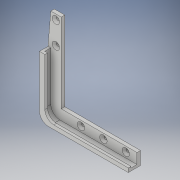
# Autodesk Inventor part: iPadGolf6HolderMount
Saved by Autodesk Inventor 2017 (Build 210142000, 142)
## iProperties
Created: 2022-11-14
Part Number: iPadGolf6HolderMount
Material: Generic
Document SubType Name: Modeling
Designer: khonsu
Density: 1 g/cm^3
Appearance: Default
Author: khonsu
Autodesk Inventor part; units mm, degrees
ref_plane "YZ Plane" through (0, 0, 0) normal (1, 0, 0) x (0, 1, 0)
ref_plane "XZ Plane" through (0, 0, 0) normal (0, 1, 0) x (-1, 0, 0)
ref_plane "XY Plane" through (0, 0, 0) normal (0, 0, 1) x (1, 0, 0)
sketch "Sketch1" plane through (0, 0, 0) normal (0, 0, 1) x (1, 0, 0)
  circle A0 centre (120.7, -158.2779) radius 1.75
  circle A1 centre (95.7, -158.2779) radius 1.75
  circle A2 centre (70.7, -158.2779) radius 1.75
  circle A3 centre (17.5, -69.45) radius 1.75
  circle A4 centre (17.5, -94.45) radius 1.75
  line L0 (135.7, -152.5058) -> (135.7, -164.0501) construction
  circle A5 centre (45.7, -158.2779) radius 1.75
  line L1 (0, 0) -> (135.7, 0) construction
  line L2 (135.7, 0) -> (135.7, -9.1902) construction
  circle A6 centre (125.7, -4.5951) radius 1.75 construction
  circle A7 centre (115.7, -4.5951) radius 1.75 construction
  line L3 (-18.071, -149.5998) -> (178.1747, -149.5998) construction
  line L4 (23.9, 14.4501) -> (135.7, 14.4501)
  line L5 (135.7, 14.4501) -> (135.7, -164.0499)
  line L6 (135.7, -164.0499) -> (23.9, -164.0499)
  line L7 (11.9, -152.0499) -> (11.9, 2.4501)
  arc A8 (23.9, 14.4501) -> (11.9, 2.4501) centre (23.9, 2.4501) ccw
  arc A9 (11.9, -152.0499) -> (23.9, -164.0499) centre (23.9, -152.0499) ccw construction
  line L8 (11.9, -20.5499) -> (8.9, -20.5499)
  line L9 (8.9, -20.5499) -> (8.9, -164.0499)
  line L10 (8.9, -164.0499) -> (11.9, -164.0499)
  line L11 (11.9, -154.0499) -> (11.9, -20.5499)
  line L12 (8.9, -55.2999) -> (11.9, -55.2999)
  line L13 (11.9, -55.2999) -> (11.9, -94.2999)
  line L14 (11.9, -94.2999) -> (8.9, -94.2999)
  line L15 (8.9, -94.2999) -> (8.9, -55.2999)
  line L16 (21.9, -164.0499) -> (135.7, -164.0499)
  line L17 (135.7, -164.0499) -> (135.7, -167.0499)
  line L18 (135.7, -167.0499) -> (8.9, -167.0499)
  line L19 (8.9, -167.0499) -> (8.9, -164.0499)
  arc A10 (11.9, -154.0499) -> (21.9, -164.0499) centre (21.9, -154.0499) ccw
  line L20 (8.9, -20.5499) -> (23.5, -20.5499)
  line L21 (23.5, -167.0499) -> (8.9, -167.0499)
  line L22 (8.9, -167.0499) -> (8.9, -20.5499)
  line L23 (135.7, -138.0558) -> (135.7, -164.0499)
  line L24 (135.7, -164.0499) -> (11.9, -164.0499)
  line L25 (11.9, -164.0499) -> (11.9, -138.0558)
  line L26 (23.5, -20.5499) -> (23.5, -138.0558)
  line L27 (23.5, -149.5998) -> (23.5, -167.0499)
  line L28 (130.7, -138.0558) -> (130.7, -167.0499)
  line L29 (130.7, -167.0499) -> (135.7, -167.0499)
  line L30 (135.7, -167.0499) -> (135.7, -138.0558)
  line L31 (-26.1104, -138.0558) -> (23.5, -138.0558) construction
  line L32 (135.7, -138.0558) -> (178.6938, -138.0558) construction
  circle A11 centre (118.0205, -143.8278) radius 1.75 construction
  line L33 (130.7, -138.0558) -> (130.7, -152.5059)
  line L34 (130.7, -152.5059) -> (23.5, -152.5059)
  line L35 (23.5, -152.5059) -> (23.5, -138.0558)
  point P0 (20.72, -105.8556)
  point P1 (11.9, -164.0499)
  dimension "d0" = 3.5
  dimension "d1" = 3.5
  dimension "d2" = 3.5
  dimension "d3" = 3.5
  dimension "d4" = 3.5
  dimension "d5" = 15
  dimension "d6" = 25
  dimension "d7" = 25
  dimension "d8" = 3.5
  dimension "d9" = 25
  dimension "d10" = 69.45
  dimension "d11" = 25
  dimension "d13" = 3.5
  dimension "d14" = 3.5
  dimension "d15" = 10
  dimension "d16" = 10
  dimension "d17" = 17.5
  dimension "d18" = 0
  dimension "d20" = 123.8
  dimension "d21" = 178.5
  dimension "d22" = 149.5999
  dimension "d23" = 12
  dimension "d26" = 14.4501
  dimension "d27" = 0
  dimension "d28" = 0
  dimension "d29" = 135.7
  dimension "d30" = 3
  dimension "d31" = 35
  dimension "d32" = 0
  dimension "d33" = 3
  dimension "d34" = 39
  dimension "d35" = 69.75
  dimension "d36" = 3
  dimension "d37" = 0
  dimension "d38" = 10
  dimension "d46" = 5
  dimension "d72" = 5.772
  dimension "d73" = 3.5
  dimension "d74" = 5.772
  dimension "d75" = 14.4501
  dimension "d76" = 5.772
  constraints: 72 end point, 14 parallel, 12 centre point, 12 point on line, 8 horizontal, 6 perpendicular, 6 point on circle, 6 tangent, 1 equal radius
  measures "d0" diameter of A0
  measures "d1" diameter of A1
  measures "d2" diameter of A2
  measures "d3" diameter of A3
  measures "d4" diameter of A4
  measures "d5" distance from line of L0 A0.centre
  measures "d6" distance of A0.centre A1.centre
  measures "d7" distance of A1.centre A2.centre
  measures "d8" diameter of A5
  measures "d9" distance of A2.centre A5.centre
  measures "d10" distance from line of L1 A3.centre
  measures "d11" distance of A3.centre A4.centre
  measures "d13" diameter of A6
  measures "d14" diameter of A7
  measures "d15" distance from line of L2 A6.centre
  measures "d16" distance of A6.centre A7.centre
  measures "d17" horizontal distance of L1.start A3.centre
  measures "d18" horizontal distance of A3.centre A4.centre
  measures "d20" distance of L5.end point (11.9, -164.05)
  measures "d21" distance of L4.end L5.end
  measures "d22" distance between parallel lines of L3 L1
  measures "d23" radius of A8
  measures "d26" distance between parallel lines of L1 L4
  measures "d27" distance from line of point (0, 0) L1
  measures "d28" distance between parallel lines of L2 L5
  measures "d29" distance from line of point (0, 0) L2
  measures "d30" distance of L10.end L9.end
  measures "d31" distance between parallel lines of L4 L8
  measures "d32" distance between parallel lines of L6 L10
  measures "d33" distance of L13.end L14.end
  measures "d34" distance of L12.end L13.end
  measures "d35" distance between parallel lines of L4 L12
  measures "d36" distance of L16.end L17.end
  measures "d37" distance between parallel lines of L5 L17
  measures "d38" radius of A10
  measures "d46" distance of L29.end L28.end
  measures "d72" distance from line of L6 A0.centre
  measures "d73" diameter of A11
  measures "d74" distance from line of L3 A11.centre
  measures "d75" vertical distance of A0.centre A11.centre
  measures "d76" distance from line of A0.centre L34
extrude "Extrusion1" add sketch "Sketch1" along normal blind 4 contours A0 | L20 L26 L35 L27 L16 A10 L11 L7 | L7 L12 L9 L8 | L28 L18 L27 L16 L6 | L6 L16 L27 L34 L28 | L7 L11 L25 L10 L9 L14 | L27 L18 L19 L10 L24 L16 | L24 L25 A10
chamfer "Chamfer1" distance 2.4 angle 45 5 edges at (15.75, -69.45, 4) (15.75, -94.45, 4) (43.95, -158.2779, 4) (68.95, -158.2779, 4) (93.95, -158.2779, 4)
sketch "Sketch2" plane through (0, 0, 4) normal (0, 0, 1) x (1, 0, 0)
  line L0 (8.9, -20.5499) -> (8.9, -55.2999) projected
  line L1 (11.9, -94.2999) -> (11.9, -55.2999) projected
  line L2 (8.9, -20.5499) -> (11.9, -20.5499)
  line L3 (11.9, -20.5499) -> (11.9, -55.2999)
  line L4 (11.9, -55.2999) -> (8.9, -55.2999)
  line L5 (8.9, -55.2999) -> (8.9, -20.5499)
  line L6 (8.9, -94.2999) -> (8.9, -167.0499) projected
  line L7 (8.9, -167.0499) -> (130.7, -167.0499) projected
  line L8 (8.9, -94.2999) -> (11.9, -94.2999)
  line L9 (11.9, -94.2999) -> (11.9, -167.0499)
  line L10 (11.9, -167.0499) -> (8.9, -167.0499)
  line L11 (8.9, -167.0499) -> (8.9, -94.2999)
  line L12 (130.7, -167.0499) -> (11.9, -167.0499)
  line L13 (11.9, -167.0499) -> (11.9, -164.0499)
  line L14 (11.9, -164.0499) -> (130.7, -164.0499)
  line L15 (130.7, -164.0499) -> (130.7, -167.0499)
  point P0 (0, 0)
  dimension "d47" = 3
  constraints: 24 end point, 6 parallel, 3 horizontal, 3 perpendicular, 3 point on line
  measures "d47" distance of L12.end L13.end
extrude "Extrusion2" add sketch "Sketch2" along normal blind 9.7
sketch "Sketch3" plane through (0, 0, 13.7) normal (0, 0, 1) x (1, 0, 0)
  line L0 (8.9, -94.2999) -> (8.9, -167.0499) projected
  line L1 (8.9, -167.0499) -> (130.7, -167.0499) projected
  line L2 (8.9, -94.2999) -> (14.9, -94.2999)
  line L3 (14.9, -94.2999) -> (14.9, -152.5499)
  line L4 (14.9, -167.0499) -> (8.9, -167.0499)
  line L5 (8.9, -167.0499) -> (8.9, -94.2999)
  line L6 (130.7, -167.0499) -> (14.9, -167.0499)
  line L7 (14.9, -167.0499) -> (14.9, -162.5499)
  line L8 (24.9, -162.5499) -> (130.7, -162.5499)
  line L9 (130.7, -162.5499) -> (130.7, -167.0499)
  line L10 (8.9, -20.5499) -> (8.9, -55.2999) projected
  line L11 (8.9, -20.5499) -> (14.9, -20.5499)
  line L12 (14.9, -20.5499) -> (14.9, -55.2999)
  line L13 (14.9, -55.2999) -> (8.9, -55.2999)
  line L14 (8.9, -55.2999) -> (8.9, -20.5499)
  arc A0 (14.9, -152.5499) -> (24.9, -162.5499) centre (24.9, -152.5499) ccw
  point P0 (0, 0)
  dimension "d50" = 6
  dimension "d51" = 4.5
  dimension "d52" = 6
  dimension "d53" = 10
  constraints: 24 end point, 6 parallel, 4 point on line, 3 horizontal, 3 perpendicular, 2 point on circle, 2 tangent, 1 centre point
  measures "d50" distance of L4.start L4.end
  measures "d51" distance of L6.end L7.end
  measures "d52" distance of L12.end L13.end
  measures "d53" radius of A0
extrude "Extrusion3" add sketch "Sketch3" against normal blind 3
sketch "Sketch4" plane through (0, 0, 13.7) normal (0, 0, 1) x (1, 0, 0)
  line L0 (130.7, -164.0499) -> (130.7, -152.5059) projected
  line L1 (130.7, -138.0558) -> (108.2, -138.0558)
  line L2 (108.2, -138.0558) -> (108.2, -174.4864)
  line L3 (108.2, -174.4864) -> (130.7, -174.4864)
  line L4 (130.7, -174.4864) -> (130.7, -138.0558)
  line L5 (-4.6471, -18.4715) -> (48.1424, -18.4715)
  line L6 (48.1424, -18.4715) -> (48.1424, -63.678)
  line L7 (48.1424, -63.678) -> (-4.6471, -63.678)
  line L8 (-4.6471, -63.678) -> (-4.6471, -18.4715)
  circle A0 centre (17.5, -69.45) radius 4.15 projected
  circle A1 centre (17.5, -69.45) radius 0.7081
  point P0 (0, 0)
  dimension "d62" = 22.5
  dimension "d79" = 5.772
  constraints: 16 end point, 4 parallel, 2 horizontal, 2 perpendicular, 1 centre point, 1 coincident
  measures "d62" distance between parallel lines of L0 L2
  measures "d79" distance from line of L7 A1.centre
extrude "Extrusion5" cut sketch "Sketch4" against normal blind 22.05 contours L4 L3 L2 L1 L0 | L5 L6 L7 L8
sketch "Sketch5" plane through (0, 0, 13.7) normal (0, 0, 1) x (1, 0, 0)
  line L0 (-3.6304, -50.2999) -> (31.4299, -50.2999)
  line L1 (31.4299, -50.2999) -> (31.4299, -99.2999)
  line L2 (31.4299, -99.2999) -> (-3.6304, -99.2999)
  line L3 (-3.6304, -99.2999) -> (-3.6304, -50.2999)
  line L4 (8.9, -55.2999) -> (14.9, -55.2999) projected
  line L5 (14.9, -94.2999) -> (8.9, -94.2999) projected
  point P0 (0, 0)
  dimension "d67" = 5
  dimension "d68" = 5
  constraints: 8 end point, 2 parallel, 1 horizontal, 1 perpendicular
  measures "d67" distance between parallel lines of L4 L0
  measures "d68" distance between parallel lines of L5 L2
extrude "Extrusion6" cut sketch "Sketch5" against normal up to surface (9.7 mm away)
fillet "Fillet1" radius 10 1 edges at (8.9, -167.0499, 6.85)
fillet "Fillet2" radius 10 1 edges at (11.9, -164.0499, 7.35)
chamfer "Chamfer3" distance 3 angle 45 1 edges at (8.9, -94.2999, 2)
sketch "Sketch6" plane through (0, 0, 4) normal (0, 0, 1) x (1, 0, 0)
  line L0 (11.9, -63.678) -> (11.9, -94.2999) projected
  line L1 (8.9, -97.2999) -> (11.9, -94.2999) projected
  line L2 (11.9, -63.678) -> (8.9, -97.2999)
  line L3 (8.9, -97.2999) -> (11.9, -94.2999)
  line L4 (11.9, -94.2999) -> (11.9, -63.678)
  point P0 (0, 0)
  constraints: 6 end point, 1 point on line, 1 vertical
extrude "Extrusion7" add sketch "Sketch6" against normal up to surface (4 mm away)
equation "\"d26\" = -0.5 * d22 + 0.5 * d21"
equation "\"d35\" = -0.5 * d34 + 0.5 * d21"
equation "\"d39\" = d19"
equation "\"d19\" = 5.772"
body "Solid1"
